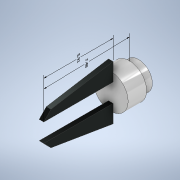
# Autodesk Inventor part: Grip
Saved by Autodesk Inventor 2022 (Build 260153000, 153)
## iProperties
Created: 2021-10-29
Part Number: Grip
Material: Generic
Document SubType Name: Modeling
Designer: Mark Maara
Density: 1 g/cm^3
Appearance: Aluminum - Polished
Mass: 269.835 g
Surface Area: 465.881 cm^2
Volume: 269.835 cm^3
Author: Mark Maara
Autodesk Inventor part; units mm, degrees
ref_plane "YZ Plane" through (0, 0, 0) normal (1, 0, 0) x (0, 1, 0)
ref_plane "XZ Plane" through (0, 0, 0) normal (0, 1, 0) x (-1, 0, 0)
ref_plane "XY Plane" through (0, 0, 0) normal (0, 0, 1) x (1, 0, 0)
sketch "Sketch1" plane through (0, 0, 0) normal (0, 0, 1) x (1, 0, 0)
  circle A0 centre (0, 0) radius 37.5
  dimension "d0" = 75
  constraints: 1 centre point, 1 coincident
  measures "d0" diameter of A0
extrude "Extrusion1" add sketch "Sketch1" along normal blind 40
sketch "Sketch2" plane through (0, 0, 0) normal (0, 0, -1) x (-1, 0, 0)
  circle A0 centre (0, 0) radius 30
  circle A1 centre (-1.5403, 0) radius 25
  dimension "d3" = 60
  dimension "d4" = 50
  constraints: 2 centre point, 1 coincident
  measures "d3" diameter of A0
  measures "d4" diameter of A1
extrude "Extrusion2" add sketch "Sketch2" along normal blind 20
sketch "Sketch3" plane through (0, 0, 0) normal (1, 0, 0) x (0, 1, 0)
  line L0 (37.5, 40) -> (-37.5, 40) projected
  line L1 (20, 40) -> (58.4777, 40)
  line L2 (20, 190) -> (20, 40)
  line L3 (58.4777, 40) -> (36.0386, 174.5807)
  line L4 (36.0386, 174.5807) -> (20, 190)
  line L5 (0, 40) -> (0, 219.4049)
  line L6 (-20, 40) -> (-58.4777, 40)
  line L7 (-20, 190) -> (-20, 40)
  line L8 (-58.4777, 40) -> (-36.0386, 174.5807)
  line L9 (-36.0386, 174.5807) -> (-20, 190)
  point P0 (0, 0)
  dimension "d8" = 150
  dimension "d11" = 40
  constraints: 18 end point, 4 symmetric about line, 1 horizontal, 1 midpoint, 1 point on line, 1 vertical
  measures "d8" distance of L2.start L1.start
  measures "d11" distance between parallel lines of L7 L2
extrude "Extrusion3" add sketch "Sketch3" along normal mid plane 10
body "Solid1"
